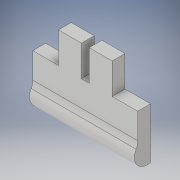
# Autodesk Inventor part: batteryFalg
Saved by Autodesk Inventor 2018.2 (Build 222227000, 227)
## iProperties
Created: 2019-03-07
Part Number: batteryFalg
Material: Generic
Document SubType Name: Modeling
Designer: ishaa
Density: 1 g/cm^3
Appearance: Default
Author: ishaa
Autodesk Inventor part; units mm, degrees
ref_plane "YZ Plane" through (0, 0, 0) normal (1, 0, 0) x (0, 1, 0)
ref_plane "XZ Plane" through (0, 0, 0) normal (0, 1, 0) x (-1, 0, 0)
ref_plane "XY Plane" through (0, 0, 0) normal (0, 0, 1) x (1, 0, 0)
sketch "Sketch1" plane through (0, 0, 0) normal (0, 1, 0) x (-1, 0, 0)
  line L0 (-6.6675, 1.5875) -> (6.6675, 1.5875)
  line L1 (6.6675, 1.5875) -> (6.6675, -1.5875)
  line L2 (6.6675, -1.5875) -> (-6.6675, -1.5875)
  line L3 (-6.6675, -1.5875) -> (-6.6675, 1.5875)
  point P0 (0, 0)
  dimension "d0" = 13.335
  dimension "d1" = 3.175
  dimension "d2" = 1.5875
  dimension "d3" = 6.6675
  constraints: 8 end point, 2 parallel, 1 horizontal, 1 perpendicular
  measures "d0" distance of L1.end L2.end
  measures "d1" distance between parallel lines of L2 L0
  measures "d2" distance from line of point (0, 0) L2
  measures "d3" distance from line of point (0, 0) L1
extrude "Extrusion1" add sketch "Sketch1" along normal blind 12.7
sketch "Sketch2" plane through (0, 12.7, 0) normal (0, 1, 0) x (1, 0, 0)
  line L0 (6.6675, -1.5875) -> (6.6675, 1.5875) projected
  line L1 (6.6675, 1.5875) -> (-6.6675, 1.5875) projected
  line L2 (-6.6675, 1.5875) -> (-6.6675, -1.5875) projected
  line L3 (-6.6675, -1.5875) -> (-0.9525, -1.5875)
  line L4 (-0.9525, -1.5875) -> (-0.9525, 1.5875)
  line L5 (-0.9525, 1.5875) -> (-6.6675, 1.5875)
  line L6 (-6.6675, 1.5875) -> (-6.6675, -1.5875)
  line L7 (6.6675, -1.5875) -> (0.9525, -1.5875)
  line L8 (0.9525, -1.5875) -> (0.9525, 1.5875)
  line L9 (0.9525, 1.5875) -> (6.6675, 1.5875)
  line L10 (6.6675, 1.5875) -> (6.6675, -1.5875)
  point P0 (0, 0)
  dimension "d6" = 5.715
  dimension "d7" = 5.715
  constraints: 16 end point, 4 parallel, 2 horizontal, 2 perpendicular, 2 point on line
  measures "d6" distance between parallel lines of L2 L4
  measures "d7" distance between parallel lines of L0 L8
extrude "Extrusion2" add sketch "Sketch2" along normal blind 7.62
sketch "Sketch3" plane through (6.6675, 0, 1.5875) normal (1, 0, 0) x (0, 0, -1)
  line L0 (3.175, 0) -> (0, 0) projected
  line L1 (3.175, 0) -> (3.175, 20.32) projected
  line L2 (0, 0) -> (3.175, 0)
  line L3 (3.175, 0) -> (3.175, 12.7)
  line L4 (3.175, 12.7) -> (0, 12.7)
  line L5 (0, 12.7) -> (0, 0)
  point P0 (1.5875, 0)
  dimension "d10" = 0
  dimension "d11" = 12.7
  constraints: 8 end point, 2 parallel, 1 horizontal, 1 perpendicular
  measures "d10" distance between parallel lines of L1 L3
  measures "d11" distance between parallel lines of L0 L4
extrude "Extrusion3" add sketch "Sketch3" along normal blind 6.35
sketch "Sketch4" plane through (-6.6675, 0, -1.5875) normal (-1, 0, 0) x (0, 0, 1)
  line L0 (0, 0) -> (3.175, 0)
  line L1 (3.175, 0) -> (3.175, 12.7)
  line L2 (3.175, 12.7) -> (0, 12.7)
  line L3 (0, 12.7) -> (0, 0)
  point P0 (1.5875, 0)
  dimension "d14" = 3.175
  dimension "d15" = 12.7
  constraints: 8 end point, 2 parallel, 1 horizontal, 1 perpendicular
  measures "d14" distance of L2.end L1.end
  measures "d15" distance of L1.end L0.end
extrude "Extrusion4" add sketch "Sketch4" along normal blind 6.35
sketch "Sketch5" plane through (0.9525, 20.32, 1.5875) normal (0, 0, 1) x (1, 0, 0)
  line L0 (-13.97, -20.32) -> (12.065, -20.32)
  line L1 (12.065, -20.32) -> (12.065, -17.145)
  line L2 (12.065, -17.145) -> (-13.97, -17.145)
  line L3 (-13.97, -17.145) -> (-13.97, -20.32)
  point P0 (-0.9525, -20.32)
  dimension "d18" = 26.035
  dimension "d19" = 3.175
  constraints: 8 end point, 2 parallel, 1 horizontal, 1 perpendicular
  measures "d18" distance of L2.end L1.end
  measures "d19" distance of L1.end L0.end
extrude "Extrusion5" add sketch "Sketch5" along normal blind 3.175
fillet "Fillet1" radius 3.175 3 edges at (0, 3.175, 4.7625) (0, 3.175, 1.5875) (0, 0, 4.7625)
equation "\"d2\" = 0.5 * d1"
equation "\"d3\" = 0.5 * d0"
equation "\"d7\" = d6"
body "Solid1"
